Autodesk Inventor part; units mm, degrees
(part 10 of 15)
  arc A4366 (-10.816, -104.5572) -> (-10.816, -104.6588) centre (-10.816, -104.608) ccw
  arc A4367 (-8.784, -104.6588) -> (-8.784, -104.5572) centre (-8.784, -104.608) ccw
  line L2010 (-10.816, -104.608) -> (-10.816, -103.592)
  arc A4368 (-10.7652, -103.592) -> (-10.8668, -103.592) centre (-10.816, -103.592) ccw
  arc A4369 (-10.8668, -104.608) -> (-10.7652, -104.608) centre (-10.816, -104.608) ccw
  line L2011 (7.584, -84.992) -> (9.616, -84.992)
  arc A4370 (9.616, -85.0428) -> (9.616, -84.9412) centre (9.616, -84.992) ccw
  arc A4371 (7.584, -84.9412) -> (7.584, -85.0428) centre (7.584, -84.992) ccw
  line L2012 (9.616, -84.992) -> (9.616, -86.008)
  arc A4372 (9.5652, -86.008) -> (9.6668, -86.008) centre (9.616, -86.008) ccw
  arc A4373 (9.6668, -84.992) -> (9.5652, -84.992) centre (9.616, -84.992) ccw
  line L2013 (9.616, -86.008) -> (7.584, -86.008)
  arc A4374 (7.584, -85.9572) -> (7.584, -86.0588) centre (7.584, -86.008) ccw
  arc A4375 (9.616, -86.0588) -> (9.616, -85.9572) centre (9.616, -86.008) ccw
  line L2014 (7.584, -86.008) -> (7.584, -84.992)
  arc A4376 (7.6348, -84.992) -> (7.5332, -84.992) centre (7.584, -84.992) ccw
  arc A4377 (7.5332, -86.008) -> (7.6348, -86.008) centre (7.584, -86.008) ccw
  line L2015 (-8.416, -105.092) -> (-6.384, -105.092)
  arc A4378 (-6.384, -105.1428) -> (-6.384, -105.0412) centre (-6.384, -105.092) ccw
  arc A4379 (-8.416, -105.0412) -> (-8.416, -105.1428) centre (-8.416, -105.092) ccw
  line L2016 (-6.384, -105.092) -> (-6.384, -106.108)
  arc A4380 (-6.4348, -106.108) -> (-6.3332, -106.108) centre (-6.384, -106.108) ccw
  arc A4381 (-6.3332, -105.092) -> (-6.4348, -105.092) centre (-6.384, -105.092) ccw
  line L2017 (-6.384, -106.108) -> (-8.416, -106.108)
  arc A4382 (-8.416, -106.0572) -> (-8.416, -106.1588) centre (-8.416, -106.108) ccw
  arc A4383 (-6.384, -106.1588) -> (-6.384, -106.0572) centre (-6.384, -106.108) ccw
  line L2018 (-8.416, -106.108) -> (-8.416, -105.092)
  arc A4384 (-8.3652, -105.092) -> (-8.4668, -105.092) centre (-8.416, -105.092) ccw
  arc A4385 (-8.4668, -106.108) -> (-8.3652, -106.108) centre (-8.416, -106.108) ccw
  line L2019 (-8.416, -107.092) -> (-6.384, -107.092)
  arc A4386 (-6.384, -107.1428) -> (-6.384, -107.0412) centre (-6.384, -107.092) ccw
  arc A4387 (-8.416, -107.0412) -> (-8.416, -107.1428) centre (-8.416, -107.092) ccw
  line L2020 (-6.384, -107.092) -> (-6.384, -108.108)
  arc A4388 (-6.4348, -108.108) -> (-6.3332, -108.108) centre (-6.384, -108.108) ccw
  arc A4389 (-6.3332, -107.092) -> (-6.4348, -107.092) centre (-6.384, -107.092) ccw
  line L2021 (-6.384, -108.108) -> (-8.416, -108.108)
  arc A4390 (-8.416, -108.0572) -> (-8.416, -108.1588) centre (-8.416, -108.108) ccw
  arc A4391 (-6.384, -108.1588) -> (-6.384, -108.0572) centre (-6.384, -108.108) ccw
  line L2022 (-8.416, -108.108) -> (-8.416, -107.092)
  arc A4392 (-8.3652, -107.092) -> (-8.4668, -107.092) centre (-8.416, -107.092) ccw
  arc A4393 (-8.4668, -108.108) -> (-8.3652, -108.108) centre (-8.416, -108.108) ccw
  line L2023 (7.192, -93.816) -> (7.192, -91.784)
  arc A4394 (7.2428, -91.784) -> (7.1412, -91.784) centre (7.192, -91.784) ccw
  arc A4395 (7.1412, -93.816) -> (7.2428, -93.816) centre (7.192, -93.816) ccw
  line L2024 (7.192, -91.784) -> (8.208, -91.784)
  arc A4396 (8.208, -91.8348) -> (8.208, -91.7332) centre (8.208, -91.784) ccw
  arc A4397 (7.192, -91.7332) -> (7.192, -91.8348) centre (7.192, -91.784) ccw
  line L2025 (8.208, -91.784) -> (8.208, -93.816)
  arc A4398 (8.1572, -93.816) -> (8.2588, -93.816) centre (8.208, -93.816) ccw
  arc A4399 (8.2588, -91.784) -> (8.1572, -91.784) centre (8.208, -91.784) ccw
  line L2026 (8.208, -93.816) -> (7.192, -93.816)
  arc A4400 (7.192, -93.7652) -> (7.192, -93.8668) centre (7.192, -93.816) ccw
  arc A4401 (8.208, -93.8668) -> (8.208, -93.7652) centre (8.208, -93.816) ccw
  line L2027 (-8.416, -108.092) -> (-6.384, -108.092)
  arc A4402 (-6.384, -108.1428) -> (-6.384, -108.0412) centre (-6.384, -108.092) ccw
  arc A4403 (-8.416, -108.0412) -> (-8.416, -108.1428) centre (-8.416, -108.092) ccw
  line L2028 (-6.384, -108.092) -> (-6.384, -109.108)
  arc A4404 (-6.4348, -109.108) -> (-6.3332, -109.108) centre (-6.384, -109.108) ccw
  arc A4405 (-6.3332, -108.092) -> (-6.4348, -108.092) centre (-6.384, -108.092) ccw
  line L2029 (-6.384, -109.108) -> (-8.416, -109.108)
  arc A4406 (-8.416, -109.0572) -> (-8.416, -109.1588) centre (-8.416, -109.108) ccw
  arc A4407 (-6.384, -109.1588) -> (-6.384, -109.0572) centre (-6.384, -109.108) ccw
  line L2030 (-8.416, -109.108) -> (-8.416, -108.092)
  arc A4408 (-8.3652, -108.092) -> (-8.4668, -108.092) centre (-8.416, -108.092) ccw
  arc A4409 (-8.4668, -109.108) -> (-8.3652, -109.108) centre (-8.416, -109.108) ccw
  line L2031 (14.184, -101.792) -> (16.216, -101.792)
  arc A4410 (16.216, -101.8428) -> (16.216, -101.7412) centre (16.216, -101.792) ccw
  arc A4411 (14.184, -101.7412) -> (14.184, -101.8428) centre (14.184, -101.792) ccw
  line L2032 (16.216, -101.792) -> (16.216, -102.808)
  arc A4412 (16.1652, -102.808) -> (16.2668, -102.808) centre (16.216, -102.808) ccw
  arc A4413 (16.2668, -101.792) -> (16.1652, -101.792) centre (16.216, -101.792) ccw
  line L2033 (16.216, -102.808) -> (14.184, -102.808)
  arc A4414 (14.184, -102.7572) -> (14.184, -102.8588) centre (14.184, -102.808) ccw
  arc A4415 (16.216, -102.8588) -> (16.216, -102.7572) centre (16.216, -102.808) ccw
  line L2034 (14.184, -102.808) -> (14.184, -101.792)
  arc A4416 (14.2348, -101.792) -> (14.1332, -101.792) centre (14.184, -101.792) ccw
  arc A4417 (14.1332, -102.808) -> (14.2348, -102.808) centre (14.184, -102.808) ccw
  line L2035 (12.184, -103.792) -> (14.216, -103.792)
  arc A4418 (14.216, -103.8428) -> (14.216, -103.7412) centre (14.216, -103.792) ccw
  arc A4419 (12.184, -103.7412) -> (12.184, -103.8428) centre (12.184, -103.792) ccw
  line L2036 (14.216, -103.792) -> (14.216, -104.808)
  arc A4420 (14.1652, -104.808) -> (14.2668, -104.808) centre (14.216, -104.808) ccw
  arc A4421 (14.2668, -103.792) -> (14.1652, -103.792) centre (14.216, -103.792) ccw
  line L2037 (14.216, -104.808) -> (12.184, -104.808)
  arc A4422 (12.184, -104.7572) -> (12.184, -104.8588) centre (12.184, -104.808) ccw
  arc A4423 (14.216, -104.8588) -> (14.216, -104.7572) centre (14.216, -104.808) ccw
  line L2038 (12.184, -104.808) -> (12.184, -103.792)
  arc A4424 (12.2348, -103.792) -> (12.1332, -103.792) centre (12.184, -103.792) ccw
  arc A4425 (12.1332, -104.808) -> (12.2348, -104.808) centre (12.184, -104.808) ccw
  line L2039 (10.316, -91.608) -> (8.284, -91.608)
  arc A4426 (8.284, -91.5572) -> (8.284, -91.6588) centre (8.284, -91.608) ccw
  arc A4427 (10.316, -91.6588) -> (10.316, -91.5572) centre (10.316, -91.608) ccw
  line L2040 (8.284, -91.608) -> (8.284, -90.592)
  arc A4428 (8.3348, -90.592) -> (8.2332, -90.592) centre (8.284, -90.592) ccw
  arc A4429 (8.2332, -91.608) -> (8.3348, -91.608) centre (8.284, -91.608) ccw
  line L2041 (8.284, -90.592) -> (10.316, -90.592)
  arc A4430 (10.316, -90.6428) -> (10.316, -90.5412) centre (10.316, -90.592) ccw
  arc A4431 (8.284, -90.5412) -> (8.284, -90.6428) centre (8.284, -90.592) ccw
  line L2042 (10.316, -90.592) -> (10.316, -91.608)
  arc A4432 (10.2652, -91.608) -> (10.3668, -91.608) centre (10.316, -91.608) ccw
  arc A4433 (10.3668, -90.592) -> (10.2652, -90.592) centre (10.316, -90.592) ccw
  line L2043 (12.208, -101.784) -> (12.208, -103.816)
  arc A4434 (12.1572, -103.816) -> (12.2588, -103.816) centre (12.208, -103.816) ccw
  arc A4435 (12.2588, -101.784) -> (12.1572, -101.784) centre (12.208, -101.784) ccw
  line L2044 (12.208, -103.816) -> (11.192, -103.816)
  arc A4436 (11.192, -103.7652) -> (11.192, -103.8668) centre (11.192, -103.816) ccw
  arc A4437 (12.208, -103.8668) -> (12.208, -103.7652) centre (12.208, -103.816) ccw
  line L2045 (11.192, -103.816) -> (11.192, -101.784)
  arc A4438 (11.2428, -101.784) -> (11.1412, -101.784) centre (11.192, -101.784) ccw
  arc A4439 (11.1412, -103.816) -> (11.2428, -103.816) centre (11.192, -103.816) ccw
  line L2046 (11.192, -101.784) -> (12.208, -101.784)
  arc A4440 (12.208, -101.8348) -> (12.208, -101.7332) centre (12.208, -101.784) ccw
  arc A4441 (11.192, -101.7332) -> (11.192, -101.8348) centre (11.192, -101.784) ccw
  line L2047 (-5.416, -107.092) -> (-3.384, -107.092)
  arc A4442 (-3.384, -107.1428) -> (-3.384, -107.0412) centre (-3.384, -107.092) ccw
  arc A4443 (-5.416, -107.0412) -> (-5.416, -107.1428) centre (-5.416, -107.092) ccw
  line L2048 (-3.384, -107.092) -> (-3.384, -108.108)
  arc A4444 (-3.4348, -108.108) -> (-3.3332, -108.108) centre (-3.384, -108.108) ccw
  arc A4445 (-3.3332, -107.092) -> (-3.4348, -107.092) centre (-3.384, -107.092) ccw
  line L2049 (-3.384, -108.108) -> (-5.416, -108.108)
  arc A4446 (-5.416, -108.0572) -> (-5.416, -108.1588) centre (-5.416, -108.108) ccw
  arc A4447 (-3.384, -108.1588) -> (-3.384, -108.0572) centre (-3.384, -108.108) ccw
  line L2050 (-5.416, -108.108) -> (-5.416, -107.092)
  arc A4448 (-5.3652, -107.092) -> (-5.4668, -107.092) centre (-5.416, -107.092) ccw
  arc A4449 (-5.4668, -108.108) -> (-5.3652, -108.108) centre (-5.416, -108.108) ccw
  line L2051 (14.184, -103.792) -> (16.216, -103.792)
  arc A4450 (16.216, -103.8428) -> (16.216, -103.7412) centre (16.216, -103.792) ccw
  arc A4451 (14.184, -103.7412) -> (14.184, -103.8428) centre (14.184, -103.792) ccw
  line L2052 (16.216, -103.792) -> (16.216, -104.808)
  arc A4452 (16.1652, -104.808) -> (16.2668, -104.808) centre (16.216, -104.808) ccw
  arc A4453 (16.2668, -103.792) -> (16.1652, -103.792) centre (16.216, -103.792) ccw
  line L2053 (16.216, -104.808) -> (14.184, -104.808)
  arc A4454 (14.184, -104.7572) -> (14.184, -104.8588) centre (14.184, -104.808) ccw
  arc A4455 (16.216, -104.8588) -> (16.216, -104.7572) centre (16.216, -104.808) ccw
  line L2054 (14.184, -104.808) -> (14.184, -103.792)
  arc A4456 (14.2348, -103.792) -> (14.1332, -103.792) centre (14.184, -103.792) ccw
  arc A4457 (14.1332, -104.808) -> (14.2348, -104.808) centre (14.184, -104.808) ccw
  line L2055 (14.208, -101.784) -> (14.208, -103.816)
  arc A4458 (14.1572, -103.816) -> (14.2588, -103.816) centre (14.208, -103.816) ccw
  arc A4459 (14.2588, -101.784) -> (14.1572, -101.784) centre (14.208, -101.784) ccw
  line L2056 (14.208, -103.816) -> (13.192, -103.816)
  arc A4460 (13.192, -103.7652) -> (13.192, -103.8668) centre (13.192, -103.816) ccw
  arc A4461 (14.208, -103.8668) -> (14.208, -103.7652) centre (14.208, -103.816) ccw
  line L2057 (13.192, -103.816) -> (13.192, -101.784)
  arc A4462 (13.2428, -101.784) -> (13.1412, -101.784) centre (13.192, -101.784) ccw
  arc A4463 (13.1412, -103.816) -> (13.2428, -103.816) centre (13.192, -103.816) ccw
  line L2058 (13.192, -101.784) -> (14.208, -101.784)
  arc A4464 (14.208, -101.8348) -> (14.208, -101.7332) centre (14.208, -101.784) ccw
  arc A4465 (13.192, -101.7332) -> (13.192, -101.8348) centre (13.192, -101.784) ccw
  line L2059 (-6.916, 46.508) -> (-4.884, 46.508)
  arc A4466 (-4.884, 46.4572) -> (-4.884, 46.5588) centre (-4.884, 46.508) ccw
  arc A4467 (-6.916, 46.5588) -> (-6.916, 46.4572) centre (-6.916, 46.508) ccw
  line L2060 (-4.884, 46.508) -> (-4.884, 45.492)
  arc A4468 (-4.9348, 45.492) -> (-4.8332, 45.492) centre (-4.884, 45.492) ccw
  arc A4469 (-4.8332, 46.508) -> (-4.9348, 46.508) centre (-4.884, 46.508) ccw
  line L2061 (-4.884, 45.492) -> (-6.916, 45.492)
  arc A4470 (-6.916, 45.5428) -> (-6.916, 45.4412) centre (-6.916, 45.492) ccw
  arc A4471 (-4.884, 45.4412) -> (-4.884, 45.5428) centre (-4.884, 45.492) ccw
  line L2062 (-6.916, 45.492) -> (-6.916, 46.508)
  arc A4472 (-6.8652, 46.508) -> (-6.9668, 46.508) centre (-6.916, 46.508) ccw
  arc A4473 (-6.9668, 45.492) -> (-6.8652, 45.492) centre (-6.916, 45.492) ccw
  line L2063 (-6.392, 38.216) -> (-6.392, 36.184)
  arc A4474 (-6.4428, 36.184) -> (-6.3412, 36.184) centre (-6.392, 36.184) ccw
  arc A4475 (-6.3412, 38.216) -> (-6.4428, 38.216) centre (-6.392, 38.216) ccw
  line L2064 (-6.392, 36.184) -> (-7.408, 36.184)
  arc A4476 (-7.408, 36.2348) -> (-7.408, 36.1332) centre (-7.408, 36.184) ccw
  arc A4477 (-6.392, 36.1332) -> (-6.392, 36.2348) centre (-6.392, 36.184) ccw
  line L2065 (-7.408, 36.184) -> (-7.408, 38.216)
  arc A4478 (-7.3572, 38.216) -> (-7.4588, 38.216) centre (-7.408, 38.216) ccw
  arc A4479 (-7.4588, 36.184) -> (-7.3572, 36.184) centre (-7.408, 36.184) ccw
  line L2066 (-7.408, 38.216) -> (-6.392, 38.216)
  arc A4480 (-6.392, 38.1652) -> (-6.392, 38.2668) centre (-6.392, 38.216) ccw
  arc A4481 (-7.408, 38.2668) -> (-7.408, 38.1652) centre (-7.408, 38.216) ccw
  line L2067 (-7.392, 38.216) -> (-7.392, 36.184)
  arc A4482 (-7.4428, 36.184) -> (-7.3412, 36.184) centre (-7.392, 36.184) ccw
  arc A4483 (-7.3412, 38.216) -> (-7.4428, 38.216) centre (-7.392, 38.216) ccw
  line L2068 (-7.392, 36.184) -> (-8.408, 36.184)
  arc A4484 (-8.408, 36.2348) -> (-8.408, 36.1332) centre (-8.408, 36.184) ccw
  arc A4485 (-7.392, 36.1332) -> (-7.392, 36.2348) centre (-7.392, 36.184) ccw
  line L2069 (-8.408, 36.184) -> (-8.408, 38.216)
  arc A4486 (-8.3572, 38.216) -> (-8.4588, 38.216) centre (-8.408, 38.216) ccw
  arc A4487 (-8.4588, 36.184) -> (-8.3572, 36.184) centre (-8.408, 36.184) ccw
  line L2070 (-8.408, 38.216) -> (-7.392, 38.216)
  arc A4488 (-7.392, 38.1652) -> (-7.392, 38.2668) centre (-7.392, 38.216) ccw
  arc A4489 (-8.408, 38.2668) -> (-8.408, 38.1652) centre (-8.408, 38.216) ccw
  line L2071 (-4.016, 39.308) -> (-1.984, 39.308)
  arc A4490 (-1.984, 39.2572) -> (-1.984, 39.3588) centre (-1.984, 39.308) ccw
  arc A4491 (-4.016, 39.3588) -> (-4.016, 39.2572) centre (-4.016, 39.308) ccw
  line L2072 (-1.984, 39.308) -> (-1.984, 38.292)
  arc A4492 (-2.0348, 38.292) -> (-1.9332, 38.292) centre (-1.984, 38.292) ccw
  arc A4493 (-1.9332, 39.308) -> (-2.0348, 39.308) centre (-1.984, 39.308) ccw
  line L2073 (-1.984, 38.292) -> (-4.016, 38.292)
  arc A4494 (-4.016, 38.3428) -> (-4.016, 38.2412) centre (-4.016, 38.292) ccw
  arc A4495 (-1.984, 38.2412) -> (-1.984, 38.3428) centre (-1.984, 38.292) ccw
  line L2074 (-4.016, 38.292) -> (-4.016, 39.308)
  arc A4496 (-3.9652, 39.308) -> (-4.0668, 39.308) centre (-4.016, 39.308) ccw
  arc A4497 (-4.0668, 38.292) -> (-3.9652, 38.292) centre (-4.016, 38.292) ccw
  line L2075 (-9.484, 40.892) -> (-11.516, 40.892)
  arc A4498 (-11.516, 40.9428) -> (-11.516, 40.8412) centre (-11.516, 40.892) ccw
  arc A4499 (-9.484, 40.8412) -> (-9.484, 40.9428) centre (-9.484, 40.892) ccw
  line L2076 (-11.516, 40.892) -> (-11.516, 41.908)
  arc A4500 (-11.4652, 41.908) -> (-11.5668, 41.908) centre (-11.516, 41.908) ccw
  arc A4501 (-11.5668, 40.892) -> (-11.4652, 40.892) centre (-11.516, 40.892) ccw
  line L2077 (-11.516, 41.908) -> (-9.484, 41.908)
  arc A4502 (-9.484, 41.8572) -> (-9.484, 41.9588) centre (-9.484, 41.908) ccw
  arc A4503 (-11.516, 41.9588) -> (-11.516, 41.8572) centre (-11.516, 41.908) ccw
  line L2078 (-9.484, 41.908) -> (-9.484, 40.892)
  arc A4504 (-9.5348, 40.892) -> (-9.4332, 40.892) centre (-9.484, 40.892) ccw
  arc A4505 (-9.4332, 41.908) -> (-9.5348, 41.908) centre (-9.484, 41.908) ccw
  line L2079 (-4.884, 44.492) -> (-6.916, 44.492)
  arc A4506 (-6.916, 44.5428) -> (-6.916, 44.4412) centre (-6.916, 44.492) ccw
  arc A4507 (-4.884, 44.4412) -> (-4.884, 44.5428) centre (-4.884, 44.492) ccw
  line L2080 (-6.916, 44.492) -> (-6.916, 45.508)
  arc A4508 (-6.8652, 45.508) -> (-6.9668, 45.508) centre (-6.916, 45.508) ccw
  arc A4509 (-6.9668, 44.492) -> (-6.8652, 44.492) centre (-6.916, 44.492) ccw
  line L2081 (-6.916, 45.508) -> (-4.884, 45.508)
  arc A4510 (-4.884, 45.4572) -> (-4.884, 45.5588) centre (-4.884, 45.508) ccw
  arc A4511 (-6.916, 45.5588) -> (-6.916, 45.4572) centre (-6.916, 45.508) ccw
  line L2082 (-4.884, 45.508) -> (-4.884, 44.492)
  arc A4512 (-4.9348, 44.492) -> (-4.8332, 44.492) centre (-4.884, 44.492) ccw
  arc A4513 (-4.8332, 45.508) -> (-4.9348, 45.508) centre (-4.884, 45.508) ccw
  line L2083 (-1.392, -88.984) -> (-1.392, -91.016)
  arc A4514 (-1.4428, -91.016) -> (-1.3412, -91.016) centre (-1.392, -91.016) ccw
  arc A4515 (-1.3412, -88.984) -> (-1.4428, -88.984) centre (-1.392, -88.984) ccw
  line L2084 (-1.392, -91.016) -> (-2.408, -91.016)
  arc A4516 (-2.408, -90.9652) -> (-2.408, -91.0668) centre (-2.408, -91.016) ccw
  arc A4517 (-1.392, -91.0668) -> (-1.392, -90.9652) centre (-1.392, -91.016) ccw
  line L2085 (-2.408, -91.016) -> (-2.408, -88.984)
  arc A4518 (-2.3572, -88.984) -> (-2.4588, -88.984) centre (-2.408, -88.984) ccw
  arc A4519 (-2.4588, -91.016) -> (-2.3572, -91.016) centre (-2.408, -91.016) ccw
  line L2086 (-2.408, -88.984) -> (-1.392, -88.984)
  arc A4520 (-1.392, -89.0348) -> (-1.392, -88.9332) centre (-1.392, -88.984) ccw
  arc A4521 (-2.408, -88.9332) -> (-2.408, -89.0348) centre (-2.408, -88.984) ccw
  line L2087 (16.284, -83.392) -> (18.316, -83.392)
  arc A4522 (18.316, -83.4428) -> (18.316, -83.3412) centre (18.316, -83.392) ccw
  arc A4523 (16.284, -83.3412) -> (16.284, -83.4428) centre (16.284, -83.392) ccw
  line L2088 (18.316, -83.392) -> (18.316, -84.408)
  arc A4524 (18.2652, -84.408) -> (18.3668, -84.408) centre (18.316, -84.408) ccw
  arc A4525 (18.3668, -83.392) -> (18.2652, -83.392) centre (18.316, -83.392) ccw
  line L2089 (18.316, -84.408) -> (16.284, -84.408)
  arc A4526 (16.284, -84.3572) -> (16.284, -84.4588) centre (16.284, -84.408) ccw
  arc A4527 (18.316, -84.4588) -> (18.316, -84.3572) centre (18.316, -84.408) ccw
  line L2090 (16.284, -84.408) -> (16.284, -83.392)
  arc A4528 (16.3348, -83.392) -> (16.2332, -83.392) centre (16.284, -83.392) ccw
  arc A4529 (16.2332, -84.408) -> (16.3348, -84.408) centre (16.284, -84.408) ccw
  line L2091 (-21.992, -6.784) -> (-21.992, -8.816)
  arc A4530 (-22.0428, -8.816) -> (-21.9412, -8.816) centre (-21.992, -8.816) ccw
  arc A4531 (-21.9412, -6.784) -> (-22.0428, -6.784) centre (-21.992, -6.784) ccw
  line L2092 (-21.992, -8.816) -> (-23.008, -8.816)
  arc A4532 (-23.008, -8.7652) -> (-23.008, -8.8668) centre (-23.008, -8.816) ccw
  arc A4533 (-21.992, -8.8668) -> (-21.992, -8.7652) centre (-21.992, -8.816) ccw
  line L2093 (-23.008, -8.816) -> (-23.008, -6.784)
  arc A4534 (-22.9572, -6.784) -> (-23.0588, -6.784) centre (-23.008, -6.784) ccw
  arc A4535 (-23.0588, -8.816) -> (-22.9572, -8.816) centre (-23.008, -8.816) ccw
  line L2094 (-23.008, -6.784) -> (-21.992, -6.784)
  arc A4536 (-21.992, -6.8348) -> (-21.992, -6.7332) centre (-21.992, -6.784) ccw
  arc A4537 (-23.008, -6.7332) -> (-23.008, -6.8348) centre (-23.008, -6.784) ccw
  line L2095 (-16.992, 16.216) -> (-16.992, 14.184)
  arc A4538 (-17.0428, 14.184) -> (-16.9412, 14.184) centre (-16.992, 14.184) ccw
  arc A4539 (-16.9412, 16.216) -> (-17.0428, 16.216) centre (-16.992, 16.216) ccw
  line L2096 (-16.992, 14.184) -> (-18.008, 14.184)
  arc A4540 (-18.008, 14.2348) -> (-18.008, 14.1332) centre (-18.008, 14.184) ccw
  arc A4541 (-16.992, 14.1332) -> (-16.992, 14.2348) centre (-16.992, 14.184) ccw
  line L2097 (-18.008, 14.184) -> (-18.008, 16.216)
  arc A4542 (-17.9572, 16.216) -> (-18.0588, 16.216) centre (-18.008, 16.216) ccw
  arc A4543 (-18.0588, 14.184) -> (-17.9572, 14.184) centre (-18.008, 14.184) ccw
  line L2098 (-18.008, 16.216) -> (-16.992, 16.216)
  arc A4544 (-16.992, 16.1652) -> (-16.992, 16.2668) centre (-16.992, 16.216) ccw
  arc A4545 (-18.008, 16.2668) -> (-18.008, 16.1652) centre (-18.008, 16.216) ccw
  line L2099 (-9.992, 8.216) -> (-9.992, 6.184)
  arc A4546 (-10.0428, 6.184) -> (-9.9412, 6.184) centre (-9.992, 6.184) ccw
  arc A4547 (-9.9412, 8.216) -> (-10.0428, 8.216) centre (-9.992, 8.216) ccw
  line L2100 (-9.992, 6.184) -> (-11.008, 6.184)
  arc A4548 (-11.008, 6.2348) -> (-11.008, 6.1332) centre (-11.008, 6.184) ccw
  arc A4549 (-9.992, 6.1332) -> (-9.992, 6.2348) centre (-9.992, 6.184) ccw
  line L2101 (-11.008, 6.184) -> (-11.008, 8.216)
  arc A4550 (-10.9572, 8.216) -> (-11.0588, 8.216) centre (-11.008, 8.216) ccw
  arc A4551 (-11.0588, 6.184) -> (-10.9572, 6.184) centre (-11.008, 6.184) ccw
  line L2102 (-11.008, 8.216) -> (-9.992, 8.216)
  arc A4552 (-9.992, 8.1652) -> (-9.992, 8.2668) centre (-9.992, 8.216) ccw
  arc A4553 (-11.008, 8.2668) -> (-11.008, 8.1652) centre (-11.008, 8.216) ccw
  line L2103 (1.008, 10.216) -> (1.008, 8.184)
  arc A4554 (0.9572, 8.184) -> (1.0588, 8.184) centre (1.008, 8.184) ccw
  arc A4555 (1.0588, 10.216) -> (0.9572, 10.216) centre (1.008, 10.216) ccw
  line L2104 (1.008, 8.184) -> (-0.008, 8.184)
  arc A4556 (-0.008, 8.2348) -> (-0.008, 8.1332) centre (-0.008, 8.184) ccw
  arc A4557 (1.008, 8.1332) -> (1.008, 8.2348) centre (1.008, 8.184) ccw
  line L2105 (-0.008, 8.184) -> (-0.008, 10.216)
  arc A4558 (0.0428, 10.216) -> (-0.0588, 10.216) centre (-0.008, 10.216) ccw
  arc A4559 (-0.0588, 8.184) -> (0.0428, 8.184) centre (-0.008, 8.184) ccw
  line L2106 (-0.008, 10.216) -> (1.008, 10.216)
  arc A4560 (1.008, 10.1652) -> (1.008, 10.2668) centre (1.008, 10.216) ccw
  arc A4561 (-0.008, 10.2668) -> (-0.008, 10.1652) centre (-0.008, 10.216) ccw
  line L2107 (-0.008, 10.184) -> (-0.008, 12.216)
  arc A4562 (0.0428, 12.216) -> (-0.0588, 12.216) centre (-0.008, 12.216) ccw
  arc A4563 (-0.0588, 10.184) -> (0.0428, 10.184) centre (-0.008, 10.184) ccw
  line L2108 (-0.008, 12.216) -> (1.008, 12.216)
  arc A4564 (1.008, 12.1652) -> (1.008, 12.2668) centre (1.008, 12.216) ccw
  arc A4565 (-0.008, 12.2668) -> (-0.008, 12.1652) centre (-0.008, 12.216) ccw
  line L2109 (1.008, 12.216) -> (1.008, 10.184)
  arc A4566 (0.9572, 10.184) -> (1.0588, 10.184) centre (1.008, 10.184) ccw
  arc A4567 (1.0588, 12.216) -> (0.9572, 12.216) centre (1.008, 12.216) ccw
  line L2110 (1.008, 10.184) -> (-0.008, 10.184)
  arc A4568 (-0.008, 10.2348) -> (-0.008, 10.1332) centre (-0.008, 10.184) ccw
  arc A4569 (1.008, 10.1332) -> (1.008, 10.2348) centre (1.008, 10.184) ccw
  line L2111 (6.016, 10.192) -> (3.984, 10.192)
  arc A4570 (3.984, 10.2428) -> (3.984, 10.1412) centre (3.984, 10.192) ccw
  arc A4571 (6.016, 10.1412) -> (6.016, 10.2428) centre (6.016, 10.192) ccw
  line L2112 (3.984, 10.192) -> (3.984, 11.208)
  arc A4572 (4.0348, 11.208) -> (3.9332, 11.208) centre (3.984, 11.208) ccw
  arc A4573 (3.9332, 10.192) -> (4.0348, 10.192) centre (3.984, 10.192) ccw
  line L2113 (3.984, 11.208) -> (6.016, 11.208)
  arc A4574 (6.016, 11.1572) -> (6.016, 11.2588) centre (6.016, 11.208) ccw
  arc A4575 (3.984, 11.2588) -> (3.984, 11.1572) centre (3.984, 11.208) ccw
  line L2114 (6.016, 11.208) -> (6.016, 10.192)
  arc A4576 (5.9652, 10.192) -> (6.0668, 10.192) centre (6.016, 10.192) ccw
  arc A4577 (6.0668, 11.208) -> (5.9652, 11.208) centre (6.016, 11.208) ccw
  line L2115 (-0.984, 0.192) -> (-3.016, 0.192)
  arc A4578 (-3.016, 0.2428) -> (-3.016, 0.1412) centre (-3.016, 0.192) ccw
  arc A4579 (-0.984, 0.1412) -> (-0.984, 0.2428) centre (-0.984, 0.192) ccw
  line L2116 (-3.016, 0.192) -> (-3.016, 1.208)
  arc A4580 (-2.9652, 1.208) -> (-3.0668, 1.208) centre (-3.016, 1.208) ccw
  arc A4581 (-3.0668, 0.192) -> (-2.9652, 0.192) centre (-3.016, 0.192) ccw
  line L2117 (-3.016, 1.208) -> (-0.984, 1.208)
  arc A4582 (-0.984, 1.1572) -> (-0.984, 1.2588) centre (-0.984, 1.208) ccw
  arc A4583 (-3.016, 1.2588) -> (-3.016, 1.1572) centre (-3.016, 1.208) ccw
  line L2118 (-0.984, 1.208) -> (-0.984, 0.192)
  arc A4584 (-1.0348, 0.192) -> (-0.9332, 0.192) centre (-0.984, 0.192) ccw
  arc A4585 (-0.9332, 1.208) -> (-1.0348, 1.208) centre (-0.984, 1.208) ccw
  line L2119 (-2.008, -6.816) -> (-2.008, -4.784)
  arc A4586 (-1.9572, -4.784) -> (-2.0588, -4.784) centre (-2.008, -4.784) ccw
  arc A4587 (-2.0588, -6.816) -> (-1.9572, -6.816) centre (-2.008, -6.816) ccw
  line L2120 (-2.008, -4.784) -> (-0.992, -4.784)
  arc A4588 (-0.992, -4.8348) -> (-0.992, -4.7332) centre (-0.992, -4.784) ccw
  arc A4589 (-2.008, -4.7332) -> (-2.008, -4.8348) centre (-2.008, -4.784) ccw
  line L2121 (-0.992, -4.784) -> (-0.992, -6.816)
  arc A4590 (-1.0428, -6.816) -> (-0.9412, -6.816) centre (-0.992, -6.816) ccw
  arc A4591 (-0.9412, -4.784) -> (-1.0428, -4.784) centre (-0.992, -4.784) ccw
  line L2122 (-0.992, -6.816) -> (-2.008, -6.816)
  arc A4592 (-2.008, -6.7652) -> (-2.008, -6.8668) centre (-2.008, -6.816) ccw
  arc A4593 (-0.992, -6.8668) -> (-0.992, -6.7652) centre (-0.992, -6.816) ccw
  line L2123 (1.016, 7.192) -> (-1.016, 7.192)
  arc A4594 (-1.016, 7.2428) -> (-1.016, 7.1412) centre (-1.016, 7.192) ccw
  arc A4595 (1.016, 7.1412) -> (1.016, 7.2428) centre (1.016, 7.192) ccw
  line L2124 (-1.016, 7.192) -> (-1.016, 8.208)
  arc A4596 (-0.9652, 8.208) -> (-1.0668, 8.208) centre (-1.016, 8.208) ccw
  arc A4597 (-1.0668, 7.192) -> (-0.9652, 7.192) centre (-1.016, 7.192) ccw
  line L2125 (-1.016, 8.208) -> (1.016, 8.208)
  arc A4598 (1.016, 8.1572) -> (1.016, 8.2588) centre (1.016, 8.208) ccw
  arc A4599 (-1.016, 8.2588) -> (-1.016, 8.1572) centre (-1.016, 8.208) ccw
  line L2126 (1.016, 8.208) -> (1.016, 7.192)
  arc A4600 (0.9652, 7.192) -> (1.0668, 7.192) centre (1.016, 7.192) ccw
  arc A4601 (1.0668, 8.208) -> (0.9652, 8.208) centre (1.016, 8.208) ccw
  line L2127 (2.008, 9.216) -> (2.008, 7.184)
  arc A4602 (1.9572, 7.184) -> (2.0588, 7.184) centre (2.008, 7.184) ccw
  arc A4603 (2.0588, 9.216) -> (1.9572, 9.216) centre (2.008, 9.216) ccw
  line L2128 (2.008, 7.184) -> (0.992, 7.184)
  arc A4604 (0.992, 7.2348) -> (0.992, 7.1332) centre (0.992, 7.184) ccw
  arc A4605 (2.008, 7.1332) -> (2.008, 7.2348) centre (2.008, 7.184) ccw
  line L2129 (0.992, 7.184) -> (0.992, 9.216)
  arc A4606 (1.0428, 9.216) -> (0.9412, 9.216) centre (0.992, 9.216) ccw
  arc A4607 (0.9412, 7.184) -> (1.0428, 7.184) centre (0.992, 7.184) ccw
  line L2130 (0.992, 9.216) -> (2.008, 9.216)
  arc A4608 (2.008, 9.1652) -> (2.008, 9.2668) centre (2.008, 9.216) ccw
  arc A4609 (0.992, 9.2668) -> (0.992, 9.1652) centre (0.992, 9.216) ccw
  line L2131 (-0.016, 7.208) -> (2.016, 7.208)
  arc A4610 (2.016, 7.1572) -> (2.016, 7.2588) centre (2.016, 7.208) ccw
  arc A4611 (-0.016, 7.2588) -> (-0.016, 7.1572) centre (-0.016, 7.208) ccw
  line L2132 (2.016, 7.208) -> (2.016, 6.192)
  arc A4612 (1.9652, 6.192) -> (2.0668, 6.192) centre (2.016, 6.192) ccw
  arc A4613 (2.0668, 7.208) -> (1.9652, 7.208) centre (2.016, 7.208) ccw
  line L2133 (2.016, 6.192) -> (-0.016, 6.192)
  arc A4614 (-0.016, 6.2428) -> (-0.016, 6.1412) centre (-0.016, 6.192) ccw
  arc A4615 (2.016, 6.1412) -> (2.016, 6.2428) centre (2.016, 6.192) ccw
  line L2134 (-0.016, 6.192) -> (-0.016, 7.208)
  arc A4616 (0.0348, 7.208) -> (-0.0668, 7.208) centre (-0.016, 7.208) ccw
  arc A4617 (-0.0668, 6.192) -> (0.0348, 6.192) centre (-0.016, 6.192) ccw
  line L2135 (-1.016, 6.208) -> (1.016, 6.208)
  arc A4618 (1.016, 6.1572) -> (1.016, 6.2588) centre (1.016, 6.208) ccw
  arc A4619 (-1.016, 6.2588) -> (-1.016, 6.1572) centre (-1.016, 6.208) ccw
  line L2136 (1.016, 6.208) -> (1.016, 5.192)
  arc A4620 (0.9652, 5.192) -> (1.0668, 5.192) centre (1.016, 5.192) ccw
  arc A4621 (1.0668, 6.208) -> (0.9652, 6.208) centre (1.016, 6.208) ccw
  line L2137 (1.016, 5.192) -> (-1.016, 5.192)
  arc A4622 (-1.016, 5.2428) -> (-1.016, 5.1412) centre (-1.016, 5.192) ccw
  arc A4623 (1.016, 5.1412) -> (1.016, 5.2428) centre (1.016, 5.192) ccw
  line L2138 (-1.016, 5.192) -> (-1.016, 6.208)
  arc A4624 (-0.9652, 6.208) -> (-1.0668, 6.208) centre (-1.016, 6.208) ccw
  arc A4625 (-1.0668, 5.192) -> (-0.9652, 5.192) centre (-1.016, 5.192) ccw
  line L2139 (-13.892, -20.684) -> (-13.892, -22.716)
  arc A4626 (-13.9428, -22.716) -> (-13.8412, -22.716) centre (-13.892, -22.716) ccw
  arc A4627 (-13.8412, -20.684) -> (-13.9428, -20.684) centre (-13.892, -20.684) ccw
  line L2140 (-13.892, -22.716) -> (-14.908, -22.716)
  arc A4628 (-14.908, -22.6652) -> (-14.908, -22.7668) centre (-14.908, -22.716) ccw
  arc A4629 (-13.892, -22.7668) -> (-13.892, -22.6652) centre (-13.892, -22.716) ccw
  line L2141 (-14.908, -22.716) -> (-14.908, -20.684)
  arc A4630 (-14.8572, -20.684) -> (-14.9588, -20.684) centre (-14.908, -20.684) ccw
  arc A4631 (-14.9588, -22.716) -> (-14.8572, -22.716) centre (-14.908, -22.716) ccw
  line L2142 (-14.908, -20.684) -> (-13.892, -20.684)
  arc A4632 (-13.892, -20.7348) -> (-13.892, -20.6332) centre (-13.892, -20.684) ccw
  arc A4633 (-14.908, -20.6332) -> (-14.908, -20.7348) centre (-14.908, -20.684) ccw
  line L2143 (-7.992, 2.216) -> (-7.992, 0.184)
  arc A4634 (-8.0428, 0.184) -> (-7.9412, 0.184) centre (-7.992, 0.184) ccw
  arc A4635 (-7.9412, 2.216) -> (-8.0428, 2.216) centre (-7.992, 2.216) ccw
  line L2144 (-7.992, 0.184) -> (-9.008, 0.184)
  arc A4636 (-9.008, 0.2348) -> (-9.008, 0.1332) centre (-9.008, 0.184) ccw
  arc A4637 (-7.992, 0.1332) -> (-7.992, 0.2348) centre (-7.992, 0.184) ccw
  line L2145 (-9.008, 0.184) -> (-9.008, 2.216)
  arc A4638 (-8.9572, 2.216) -> (-9.0588, 2.216) centre (-9.008, 2.216) ccw
  arc A4639 (-9.0588, 0.184) -> (-8.9572, 0.184) centre (-9.008, 0.184) ccw
  line L2146 (-9.008, 2.216) -> (-7.992, 2.216)
  arc A4640 (-7.992, 2.1652) -> (-7.992, 2.2668) centre (-7.992, 2.216) ccw
  arc A4641 (-9.008, 2.2668) -> (-9.008, 2.1652) centre (-9.008, 2.216) ccw
  line L2147 (-6.992, 2.216) -> (-6.992, 0.184)
  arc A4642 (-7.0428, 0.184) -> (-6.9412, 0.184) centre (-6.992, 0.184) ccw
  arc A4643 (-6.9412, 2.216) -> (-7.0428, 2.216) centre (-6.992, 2.216) ccw
  line L2148 (-6.992, 0.184) -> (-8.008, 0.184)
  arc A4644 (-8.008, 0.2348) -> (-8.008, 0.1332) centre (-8.008, 0.184) ccw
  arc A4645 (-6.992, 0.1332) -> (-6.992, 0.2348) centre (-6.992, 0.184) ccw
  line L2149 (-8.008, 0.184) -> (-8.008, 2.216)
  arc A4646 (-7.9572, 2.216) -> (-8.0588, 2.216) centre (-8.008, 2.216) ccw
  arc A4647 (-8.0588, 0.184) -> (-7.9572, 0.184) centre (-8.008, 0.184) ccw
  line L2150 (-8.008, 2.216) -> (-6.992, 2.216)
  arc A4648 (-6.992, 2.1652) -> (-6.992, 2.2668) centre (-6.992, 2.216) ccw
  arc A4649 (-8.008, 2.2668) -> (-8.008, 2.1652) centre (-8.008, 2.216) ccw
  line L2151 (-6.008, -4.816) -> (-6.008, -2.784)
  arc A4650 (-5.9572, -2.784) -> (-6.0588, -2.784) centre (-6.008, -2.784) ccw
  arc A4651 (-6.0588, -4.816) -> (-5.9572, -4.816) centre (-6.008, -4.816) ccw
  line L2152 (-6.008, -2.784) -> (-4.992, -2.784)
  arc A4652 (-4.992, -2.8348) -> (-4.992, -2.7332) centre (-4.992, -2.784) ccw
  arc A4653 (-6.008, -2.7332) -> (-6.008, -2.8348) centre (-6.008, -2.784) ccw
  line L2153 (-4.992, -2.784) -> (-4.992, -4.816)
  arc A4654 (-5.0428, -4.816) -> (-4.9412, -4.816) centre (-4.992, -4.816) ccw
  arc A4655 (-4.9412, -2.784) -> (-5.0428, -2.784) centre (-4.992, -2.784) ccw
  line L2154 (-4.992, -4.816) -> (-6.008, -4.816)
  arc A4656 (-6.008, -4.7652) -> (-6.008, -4.8668) centre (-6.008, -4.816) ccw
  arc A4657 (-4.992, -4.8668) -> (-4.992, -4.7652) centre (-4.992, -4.816) ccw
  line L2155 (0.984, 4.208) -> (3.016, 4.208)
  arc A4658 (3.016, 4.1572) -> (3.016, 4.2588) centre (3.016, 4.208) ccw
  arc A4659 (0.984, 4.2588) -> (0.984, 4.1572) centre (0.984, 4.208) ccw
  line L2156 (3.016, 4.208) -> (3.016, 3.192)
  arc A4660 (2.9652, 3.192) -> (3.0668, 3.192) centre (3.016, 3.192) ccw
  arc A4661 (3.0668, 4.208) -> (2.9652, 4.208) centre (3.016, 4.208) ccw
  line L2157 (3.016, 3.192) -> (0.984, 3.192)
  arc A4662 (0.984, 3.2428) -> (0.984, 3.1412) centre (0.984, 3.192) ccw
  arc A4663 (3.016, 3.1412) -> (3.016, 3.2428) centre (3.016, 3.192) ccw
  line L2158 (0.984, 3.192) -> (0.984, 4.208)
  arc A4664 (1.0348, 4.208) -> (0.9332, 4.208) centre (0.984, 4.208) ccw
  arc A4665 (0.9332, 3.192) -> (1.0348, 3.192) centre (0.984, 3.192) ccw
  line L2159 (-1.016, 4.208) -> (1.016, 4.208)
  arc A4666 (1.016, 4.1572) -> (1.016, 4.2588) centre (1.016, 4.208) ccw
  arc A4667 (-1.016, 4.2588) -> (-1.016, 4.1572) centre (-1.016, 4.208) ccw
  line L2160 (1.016, 4.208) -> (1.016, 3.192)
  arc A4668 (0.9652, 3.192) -> (1.0668, 3.192) centre (1.016, 3.192) ccw
  arc A4669 (1.0668, 4.208) -> (0.9652, 4.208) centre (1.016, 4.208) ccw
  line L2161 (1.016, 3.192) -> (-1.016, 3.192)
  arc A4670 (-1.016, 3.2428) -> (-1.016, 3.1412) centre (-1.016, 3.192) ccw
  arc A4671 (1.016, 3.1412) -> (1.016, 3.2428) centre (1.016, 3.192) ccw
  line L2162 (-1.016, 3.192) -> (-1.016, 4.208)
  arc A4672 (-0.9652, 4.208) -> (-1.0668, 4.208) centre (-1.016, 4.208) ccw
  arc A4673 (-1.0668, 3.192) -> (-0.9652, 3.192) centre (-1.016, 3.192) ccw
  line L2163 (-2.992, 2.216) -> (-2.992, 0.184)
  arc A4674 (-3.0428, 0.184) -> (-2.9412, 0.184) centre (-2.992, 0.184) ccw
  arc A4675 (-2.9412, 2.216) -> (-3.0428, 2.216) centre (-2.992, 2.216) ccw
  line L2164 (-2.992, 0.184) -> (-4.008, 0.184)
  arc A4676 (-4.008, 0.2348) -> (-4.008, 0.1332) centre (-4.008, 0.184) ccw
  arc A4677 (-2.992, 0.1332) -> (-2.992, 0.2348) centre (-2.992, 0.184) ccw
  line L2165 (-4.008, 0.184) -> (-4.008, 2.216)
  arc A4678 (-3.9572, 2.216) -> (-4.0588, 2.216) centre (-4.008, 2.216) ccw
  arc A4679 (-4.0588, 0.184) -> (-3.9572, 0.184) centre (-4.008, 0.184) ccw
  line L2166 (-4.008, 2.216) -> (-2.992, 2.216)
  arc A4680 (-2.992, 2.1652) -> (-2.992, 2.2668) centre (-2.992, 2.216) ccw
  arc A4681 (-4.008, 2.2668) -> (-4.008, 2.1652) centre (-4.008, 2.216) ccw
  line L2167 (0.984, 3.208) -> (3.016, 3.208)
  arc A4682 (3.016, 3.1572) -> (3.016, 3.2588) centre (3.016, 3.208) ccw
  arc A4683 (0.984, 3.2588) -> (0.984, 3.1572) centre (0.984, 3.208) ccw
  line L2168 (3.016, 3.208) -> (3.016, 2.192)
  arc A4684 (2.9652, 2.192) -> (3.0668, 2.192) centre (3.016, 2.192) ccw
  arc A4685 (3.0668, 3.208) -> (2.9652, 3.208) centre (3.016, 3.208) ccw
  line L2169 (3.016, 2.192) -> (0.984, 2.192)
  arc A4686 (0.984, 2.2428) -> (0.984, 2.1412) centre (0.984, 2.192) ccw
  arc A4687 (3.016, 2.1412) -> (3.016, 2.2428) centre (3.016, 2.192) ccw
  line L2170 (0.984, 2.192) -> (0.984, 3.208)
  arc A4688 (1.0348, 3.208) -> (0.9332, 3.208) centre (0.984, 3.208) ccw
  arc A4689 (0.9332, 2.192) -> (1.0348, 2.192) centre (0.984, 2.192) ccw
  line L2171 (-1.016, 3.208) -> (1.016, 3.208)
  arc A4690 (1.016, 3.1572) -> (1.016, 3.2588) centre (1.016, 3.208) ccw
  arc A4691 (-1.016, 3.2588) -> (-1.016, 3.1572) centre (-1.016, 3.208) ccw
  line L2172 (1.016, 3.208) -> (1.016, 2.192)
  arc A4692 (0.9652, 2.192) -> (1.0668, 2.192) centre (1.016, 2.192) ccw
  arc A4693 (1.0668, 3.208) -> (0.9652, 3.208) centre (1.016, 3.208) ccw
  line L2173 (1.016, 2.192) -> (-1.016, 2.192)
  arc A4694 (-1.016, 2.2428) -> (-1.016, 2.1412) centre (-1.016, 2.192) ccw
  arc A4695 (1.016, 2.1412) -> (1.016, 2.2428) centre (1.016, 2.192) ccw
  line L2174 (-1.016, 2.192) -> (-1.016, 3.208)
  arc A4696 (-0.9652, 3.208) -> (-1.0668, 3.208) centre (-1.016, 3.208) ccw
  arc A4697 (-1.0668, 2.192) -> (-0.9652, 2.192) centre (-1.016, 2.192) ccw
  line L2175 (-7.008, 0.184) -> (-7.008, 2.216)
  arc A4698 (-6.9572, 2.216) -> (-7.0588, 2.216) centre (-7.008, 2.216) ccw
  arc A4699 (-7.0588, 0.184) -> (-6.9572, 0.184) centre (-7.008, 0.184) ccw
  line L2176 (-7.008, 2.216) -> (-5.992, 2.216)
  arc A4700 (-5.992, 2.1652) -> (-5.992, 2.2668) centre (-5.992, 2.216) ccw
  arc A4701 (-7.008, 2.2668) -> (-7.008, 2.1652) centre (-7.008, 2.216) ccw
  line L2177 (-5.992, 2.216) -> (-5.992, 0.184)
  arc A4702 (-6.0428, 0.184) -> (-5.9412, 0.184) centre (-5.992, 0.184) ccw
  arc A4703 (-5.9412, 2.216) -> (-6.0428, 2.216) centre (-5.992, 2.216) ccw
  line L2178 (-5.992, 0.184) -> (-7.008, 0.184)
  arc A4704 (-7.008, 0.2348) -> (-7.008, 0.1332) centre (-7.008, 0.184) ccw
  arc A4705 (-5.992, 0.1332) -> (-5.992, 0.2348) centre (-5.992, 0.184) ccw
  line L2179 (0.984, 2.208) -> (3.016, 2.208)
  arc A4706 (3.016, 2.1572) -> (3.016, 2.2588) centre (3.016, 2.208) ccw
  arc A4707 (0.984, 2.2588) -> (0.984, 2.1572) centre (0.984, 2.208) ccw
  line L2180 (3.016, 2.208) -> (3.016, 1.192)
  arc A4708 (2.9652, 1.192) -> (3.0668, 1.192) centre (3.016, 1.192) ccw
  arc A4709 (3.0668, 2.208) -> (2.9652, 2.208) centre (3.016, 2.208) ccw
  line L2181 (3.016, 1.192) -> (0.984, 1.192)
  arc A4710 (0.984, 1.2428) -> (0.984, 1.1412) centre (0.984, 1.192) ccw
  arc A4711 (3.016, 1.1412) -> (3.016, 1.2428) centre (3.016, 1.192) ccw
  line L2182 (0.984, 1.192) -> (0.984, 2.208)
  arc A4712 (1.0348, 2.208) -> (0.9332, 2.208) centre (0.984, 2.208) ccw
  arc A4713 (0.9332, 1.192) -> (1.0348, 1.192) centre (0.984, 1.192) ccw
  line L2183 (-1.016, 2.208) -> (1.016, 2.208)
  arc A4714 (1.016, 2.1572) -> (1.016, 2.2588) centre (1.016, 2.208) ccw
  arc A4715 (-1.016, 2.2588) -> (-1.016, 2.1572) centre (-1.016, 2.208) ccw
  line L2184 (1.016, 2.208) -> (1.016, 1.192)
  arc A4716 (0.9652, 1.192) -> (1.0668, 1.192) centre (1.016, 1.192) ccw
  arc A4717 (1.0668, 2.208) -> (0.9652, 2.208) centre (1.016, 2.208) ccw
  line L2185 (1.016, 1.192) -> (-1.016, 1.192)
  arc A4718 (-1.016, 1.2428) -> (-1.016, 1.1412) centre (-1.016, 1.192) ccw
  arc A4719 (1.016, 1.1412) -> (1.016, 1.2428) centre (1.016, 1.192) ccw
  line L2186 (-1.016, 1.192) -> (-1.016, 2.208)
  arc A4720 (-0.9652, 2.208) -> (-1.0668, 2.208) centre (-1.016, 2.208) ccw
  arc A4721 (-1.0668, 1.192) -> (-0.9652, 1.192) centre (-1.016, 1.192) ccw
  line L2187 (-9.008, -1.816) -> (-9.008, 0.216)
  arc A4722 (-8.9572, 0.216) -> (-9.0588, 0.216) centre (-9.008, 0.216) ccw
  arc A4723 (-9.0588, -1.816) -> (-8.9572, -1.816) centre (-9.008, -1.816) ccw
  line L2188 (-9.008, 0.216) -> (-7.992, 0.216)
  arc A4724 (-7.992, 0.1652) -> (-7.992, 0.2668) centre (-7.992, 0.216) ccw
  arc A4725 (-9.008, 0.2668) -> (-9.008, 0.1652) centre (-9.008, 0.216) ccw
  line L2189 (-7.992, 0.216) -> (-7.992, -1.816)
  arc A4726 (-8.0428, -1.816) -> (-7.9412, -1.816) centre (-7.992, -1.816) ccw
  arc A4727 (-7.9412, 0.216) -> (-8.0428, 0.216) centre (-7.992, 0.216) ccw
  line L2190 (-7.992, -1.816) -> (-9.008, -1.816)
  arc A4728 (-9.008, -1.7652) -> (-9.008, -1.8668) centre (-9.008, -1.816) ccw
  arc A4729 (-7.992, -1.8668) -> (-7.992, -1.7652) centre (-7.992, -1.816) ccw
  line L2191 (-9.008, -3.816) -> (-9.008, -1.784)
  arc A4730 (-8.9572, -1.784) -> (-9.0588, -1.784) centre (-9.008, -1.784) ccw
  arc A4731 (-9.0588, -3.816) -> (-8.9572, -3.816) centre (-9.008, -3.816) ccw
  line L2192 (-9.008, -1.784) -> (-7.992, -1.784)
  arc A4732 (-7.992, -1.8348) -> (-7.992, -1.7332) centre (-7.992, -1.784) ccw
  arc A4733 (-9.008, -1.7332) -> (-9.008, -1.8348) centre (-9.008, -1.784) ccw
  line L2193 (-7.992, -1.784) -> (-7.992, -3.816)
  arc A4734 (-8.0428, -3.816) -> (-7.9412, -3.816) centre (-7.992, -3.816) ccw
  arc A4735 (-7.9412, -1.784) -> (-8.0428, -1.784) centre (-7.992, -1.784) ccw
  line L2194 (-7.992, -3.816) -> (-9.008, -3.816)
  arc A4736 (-9.008, -3.7652) -> (-9.008, -3.8668) centre (-9.008, -3.816) ccw
  arc A4737 (-7.992, -3.8668) -> (-7.992, -3.7652) centre (-7.992, -3.816) ccw
  line L2195 (-8.008, -1.816) -> (-8.008, 0.216)
  arc A4738 (-7.9572, 0.216) -> (-8.0588, 0.216) centre (-8.008, 0.216) ccw
  arc A4739 (-8.0588, -1.816) -> (-7.9572, -1.816) centre (-8.008, -1.816) ccw
  line L2196 (-8.008, 0.216) -> (-6.992, 0.216)
  arc A4740 (-6.992, 0.1652) -> (-6.992, 0.2668) centre (-6.992, 0.216) ccw
  arc A4741 (-8.008, 0.2668) -> (-8.008, 0.1652) centre (-8.008, 0.216) ccw
  line L2197 (-6.992, 0.216) -> (-6.992, -1.816)
  arc A4742 (-7.0428, -1.816) -> (-6.9412, -1.816) centre (-6.992, -1.816) ccw
  arc A4743 (-6.9412, 0.216) -> (-7.0428, 0.216) centre (-6.992, 0.216) ccw
  line L2198 (-6.992, -1.816) -> (-8.008, -1.816)
  arc A4744 (-8.008, -1.7652) -> (-8.008, -1.8668) centre (-8.008, -1.816) ccw
  arc A4745 (-6.992, -1.8668) -> (-6.992, -1.7652) centre (-6.992, -1.816) ccw
  line L2199 (-8.008, -3.816) -> (-8.008, -1.784)
  arc A4746 (-7.9572, -1.784) -> (-8.0588, -1.784) centre (-8.008, -1.784) ccw
  arc A4747 (-8.0588, -3.816) -> (-7.9572, -3.816) centre (-8.008, -3.816) ccw
  line L2200 (-8.008, -1.784) -> (-6.992, -1.784)
  arc A4748 (-6.992, -1.8348) -> (-6.992, -1.7332) centre (-6.992, -1.784) ccw
  arc A4749 (-8.008, -1.7332) -> (-8.008, -1.8348) centre (-8.008, -1.784) ccw
  line L2201 (-6.992, -1.784) -> (-6.992, -3.816)
  arc A4750 (-7.0428, -3.816) -> (-6.9412, -3.816) centre (-6.992, -3.816) ccw
  arc A4751 (-6.9412, -1.784) -> (-7.0428, -1.784) centre (-6.992, -1.784) ccw
  line L2202 (-6.992, -3.816) -> (-8.008, -3.816)
  arc A4752 (-8.008, -3.7652) -> (-8.008, -3.8668) centre (-8.008, -3.816) ccw
  arc A4753 (-6.992, -3.8668) -> (-6.992, -3.7652) centre (-6.992, -3.816) ccw
  line L2203 (-10.008, -0.816) -> (-10.008, 1.216)
  arc A4754 (-9.9572, 1.216) -> (-10.0588, 1.216) centre (-10.008, 1.216) ccw
  arc A4755 (-10.0588, -0.816) -> (-9.9572, -0.816) centre (-10.008, -0.816) ccw
  line L2204 (-10.008, 1.216) -> (-8.992, 1.216)
  arc A4756 (-8.992, 1.1652) -> (-8.992, 1.2668) centre (-8.992, 1.216) ccw
  arc A4757 (-10.008, 1.2668) -> (-10.008, 1.1652) centre (-10.008, 1.216) ccw
  line L2205 (-8.992, 1.216) -> (-8.992, -0.816)
  arc A4758 (-9.0428, -0.816) -> (-8.9412, -0.816) centre (-8.992, -0.816) ccw
  arc A4759 (-8.9412, 1.216) -> (-9.0428, 1.216) centre (-8.992, 1.216) ccw
  line L2206 (-8.992, -0.816) -> (-10.008, -0.816)
  arc A4760 (-10.008, -0.7652) -> (-10.008, -0.8668) centre (-10.008, -0.816) ccw
  arc A4761 (-8.992, -0.8668) -> (-8.992, -0.7652) centre (-8.992, -0.816) ccw
  line L2207 (-10.008, -2.816) -> (-10.008, -0.784)
  arc A4762 (-9.9572, -0.784) -> (-10.0588, -0.784) centre (-10.008, -0.784) ccw
  arc A4763 (-10.0588, -2.816) -> (-9.9572, -2.816) centre (-10.008, -2.816) ccw
  line L2208 (-10.008, -0.784) -> (-8.992, -0.784)
  arc A4764 (-8.992, -0.8348) -> (-8.992, -0.7332) centre (-8.992, -0.784) ccw
  arc A4765 (-10.008, -0.7332) -> (-10.008, -0.8348) centre (-10.008, -0.784) ccw
  line L2209 (-8.992, -0.784) -> (-8.992, -2.816)
  arc A4766 (-9.0428, -2.816) -> (-8.9412, -2.816) centre (-8.992, -2.816) ccw
  arc A4767 (-8.9412, -0.784) -> (-9.0428, -0.784) centre (-8.992, -0.784) ccw
  line L2210 (-8.992, -2.816) -> (-10.008, -2.816)
  arc A4768 (-10.008, -2.7652) -> (-10.008, -2.8668) centre (-10.008, -2.816) ccw
  arc A4769 (-8.992, -2.8668) -> (-8.992, -2.7652) centre (-8.992, -2.816) ccw
  line L2211 (-7.008, -3.816) -> (-7.008, -1.784)
  arc A4770 (-6.9572, -1.784) -> (-7.0588, -1.784) centre (-7.008, -1.784) ccw
  arc A4771 (-7.0588, -3.816) -> (-6.9572, -3.816) centre (-7.008, -3.816) ccw
  line L2212 (-7.008, -1.784) -> (-5.992, -1.784)
  arc A4772 (-5.992, -1.8348) -> (-5.992, -1.7332) centre (-5.992, -1.784) ccw
  arc A4773 (-7.008, -1.7332) -> (-7.008, -1.8348) centre (-7.008, -1.784) ccw
  line L2213 (-5.992, -1.784) -> (-5.992, -3.816)
  arc A4774 (-6.0428, -3.816) -> (-5.9412, -3.816) centre (-5.992, -3.816) ccw
  arc A4775 (-5.9412, -1.784) -> (-6.0428, -1.784) centre (-5.992, -1.784) ccw
  line L2214 (-5.992, -3.816) -> (-7.008, -3.816)
  arc A4776 (-7.008, -3.7652) -> (-7.008, -3.8668) centre (-7.008, -3.816) ccw
  arc A4777 (-5.992, -3.8668) -> (-5.992, -3.7652) centre (-5.992, -3.816) ccw
  line L2215 (-7.008, -5.816) -> (-7.008, -3.784)
  arc A4778 (-6.9572, -3.784) -> (-7.0588, -3.784) centre (-7.008, -3.784) ccw
  arc A4779 (-7.0588, -5.816) -> (-6.9572, -5.816) centre (-7.008, -5.816) ccw
  line L2216 (-7.008, -3.784) -> (-5.992, -3.784)
  arc A4780 (-5.992, -3.8348) -> (-5.992, -3.7332) centre (-5.992, -3.784) ccw
  arc A4781 (-7.008, -3.7332) -> (-7.008, -3.8348) centre (-7.008, -3.784) ccw
  line L2217 (-5.992, -3.784) -> (-5.992, -5.816)
  arc A4782 (-6.0428, -5.816) -> (-5.9412, -5.816) centre (-5.992, -5.816) ccw
  arc A4783 (-5.9412, -3.784) -> (-6.0428, -3.784) centre (-5.992, -3.784) ccw
  line L2218 (-5.992, -5.816) -> (-7.008, -5.816)
  arc A4784 (-7.008, -5.7652) -> (-7.008, -5.8668) centre (-7.008, -5.816) ccw
  arc A4785 (-5.992, -5.8668) -> (-5.992, -5.7652) centre (-5.992, -5.816) ccw
  line L2219 (-6.008, -0.816) -> (-6.008, 1.216)
  arc A4786 (-5.9572, 1.216) -> (-6.0588, 1.216) centre (-6.008, 1.216) ccw
  arc A4787 (-6.0588, -0.816) -> (-5.9572, -0.816) centre (-6.008, -0.816) ccw
  line L2220 (-6.008, 1.216) -> (-4.992, 1.216)
  arc A4788 (-4.992, 1.1652) -> (-4.992, 1.2668) centre (-4.992, 1.216) ccw
  arc A4789 (-6.008, 1.2668) -> (-6.008, 1.1652) centre (-6.008, 1.216) ccw
  line L2221 (-4.992, 1.216) -> (-4.992, -0.816)
  arc A4790 (-5.0428, -0.816) -> (-4.9412, -0.816) centre (-4.992, -0.816) ccw
  arc A4791 (-4.9412, 1.216) -> (-5.0428, 1.216) centre (-4.992, 1.216) ccw
  line L2222 (-4.992, -0.816) -> (-6.008, -0.816)
  arc A4792 (-6.008, -0.7652) -> (-6.008, -0.8668) centre (-6.008, -0.816) ccw
  arc A4793 (-4.992, -0.8668) -> (-4.992, -0.7652) centre (-4.992, -0.816) ccw
  line L2223 (-14.984, -0.808) -> (-17.016, -0.808)
  arc A4794 (-17.016, -0.7572) -> (-17.016, -0.8588) centre (-17.016, -0.808) ccw
  arc A4795 (-14.984, -0.8588) -> (-14.984, -0.7572) centre (-14.984, -0.808) ccw
  line L2224 (-17.016, -0.808) -> (-17.016, 0.208)
  arc A4796 (-16.9652, 0.208) -> (-17.0668, 0.208) centre (-17.016, 0.208) ccw
  arc A4797 (-17.0668, -0.808) -> (-16.9652, -0.808) centre (-17.016, -0.808) ccw
  line L2225 (-17.016, 0.208) -> (-14.984, 0.208)
  arc A4798 (-14.984, 0.1572) -> (-14.984, 0.2588) centre (-14.984, 0.208) ccw
  arc A4799 (-17.016, 0.2588) -> (-17.016, 0.1572) centre (-17.016, 0.208) ccw
  line L2226 (-14.984, 0.208) -> (-14.984, -0.808)
  arc A4800 (-15.0348, -0.808) -> (-14.9332, -0.808) centre (-14.984, -0.808) ccw
  arc A4801 (-14.9332, 0.208) -> (-15.0348, 0.208) centre (-14.984, 0.208) ccw
  line L2227 (-22.192, -20.384) -> (-22.192, -22.416)
  arc A4802 (-22.2428, -22.416) -> (-22.1412, -22.416) centre (-22.192, -22.416) ccw
  arc A4803 (-22.1412, -20.384) -> (-22.2428, -20.384) centre (-22.192, -20.384) ccw
  line L2228 (-22.192, -22.416) -> (-23.208, -22.416)
  arc A4804 (-23.208, -22.3652) -> (-23.208, -22.4668) centre (-23.208, -22.416) ccw
  arc A4805 (-22.192, -22.4668) -> (-22.192, -22.3652) centre (-22.192, -22.416) ccw
  line L2229 (-23.208, -22.416) -> (-23.208, -20.384)
  arc A4806 (-23.1572, -20.384) -> (-23.2588, -20.384) centre (-23.208, -20.384) ccw
  arc A4807 (-23.2588, -22.416) -> (-23.1572, -22.416) centre (-23.208, -22.416) ccw
  line L2230 (-23.208, -20.384) -> (-22.192, -20.384)
  arc A4808 (-22.192, -20.4348) -> (-22.192, -20.3332) centre (-22.192, -20.384) ccw
  arc A4809 (-23.208, -20.3332) -> (-23.208, -20.4348) centre (-23.208, -20.384) ccw
  line L2231 (-23.192, -20.384) -> (-23.192, -22.416)
  arc A4810 (-23.2428, -22.416) -> (-23.1412, -22.416) centre (-23.192, -22.416) ccw
  arc A4811 (-23.1412, -20.384) -> (-23.2428, -20.384) centre (-23.192, -20.384) ccw
  line L2232 (-23.192, -22.416) -> (-24.208, -22.416)
  arc A4812 (-24.208, -22.3652) -> (-24.208, -22.4668) centre (-24.208, -22.416) ccw
  arc A4813 (-23.192, -22.4668) -> (-23.192, -22.3652) centre (-23.192, -22.416) ccw
  line L2233 (-24.208, -22.416) -> (-24.208, -20.384)
  arc A4814 (-24.1572, -20.384) -> (-24.2588, -20.384) centre (-24.208, -20.384) ccw
  arc A4815 (-24.2588, -22.416) -> (-24.1572, -22.416) centre (-24.208, -22.416) ccw
  line L2234 (-24.208, -20.384) -> (-23.192, -20.384)
  arc A4816 (-23.192, -20.4348) -> (-23.192, -20.3332) centre (-23.192, -20.384) ccw
  arc A4817 (-24.208, -20.3332) -> (-24.208, -20.4348) centre (-24.208, -20.384) ccw
  line L2235 (-24.392, -24.384) -> (-24.392, -26.416)
  arc A4818 (-24.4428, -26.416) -> (-24.3412, -26.416) centre (-24.392, -26.416) ccw
  arc A4819 (-24.3412, -24.384) -> (-24.4428, -24.384) centre (-24.392, -24.384) ccw
  line L2236 (-24.392, -26.416) -> (-25.408, -26.416)
  arc A4820 (-25.408, -26.3652) -> (-25.408, -26.4668) centre (-25.408, -26.416) ccw
  arc A4821 (-24.392, -26.4668) -> (-24.392, -26.3652) centre (-24.392, -26.416) ccw
  line L2237 (-25.408, -26.416) -> (-25.408, -24.384)
  arc A4822 (-25.3572, -24.384) -> (-25.4588, -24.384) centre (-25.408, -24.384) ccw
  arc A4823 (-25.4588, -26.416) -> (-25.3572, -26.416) centre (-25.408, -26.416) ccw
  line L2238 (-25.408, -24.384) -> (-24.392, -24.384)
  arc A4824 (-24.392, -24.4348) -> (-24.392, -24.3332) centre (-24.392, -24.384) ccw
  arc A4825 (-25.408, -24.3332) -> (-25.408, -24.4348) centre (-25.408, -24.384) ccw
  line L2239 (-25.408, -24.416) -> (-25.408, -22.384)
  arc A4826 (-25.3572, -22.384) -> (-25.4588, -22.384) centre (-25.408, -22.384) ccw
  arc A4827 (-25.4588, -24.416) -> (-25.3572, -24.416) centre (-25.408, -24.416) ccw
  line L2240 (-25.408, -22.384) -> (-24.392, -22.384)
  arc A4828 (-24.392, -22.4348) -> (-24.392, -22.3332) centre (-24.392, -22.384) ccw
  arc A4829 (-25.408, -22.3332) -> (-25.408, -22.4348) centre (-25.408, -22.384) ccw
  line L2241 (-24.392, -22.384) -> (-24.392, -24.416)
  arc A4830 (-24.4428, -24.416) -> (-24.3412, -24.416) centre (-24.392, -24.416) ccw
  arc A4831 (-24.3412, -22.384) -> (-24.4428, -22.384) centre (-24.392, -22.384) ccw
  line L2242 (-24.392, -24.416) -> (-25.408, -24.416)
  arc A4832 (-25.408, -24.3652) -> (-25.408, -24.4668) centre (-25.408, -24.416) ccw
  arc A4833 (-24.392, -24.4668) -> (-24.392, -24.3652) centre (-24.392, -24.416) ccw
  line L2243 (-3.984, -1.808) -> (-6.016, -1.808)
  arc A4834 (-6.016, -1.7572) -> (-6.016, -1.8588) centre (-6.016, -1.808) ccw
  arc A4835 (-3.984, -1.8588) -> (-3.984, -1.7572) centre (-3.984, -1.808) ccw
  line L2244 (-6.016, -1.808) -> (-6.016, -0.792)
  arc A4836 (-5.9652, -0.792) -> (-6.0668, -0.792) centre (-6.016, -0.792) ccw
  arc A4837 (-6.0668, -1.808) -> (-5.9652, -1.808) centre (-6.016, -1.808) ccw
  line L2245 (-6.016, -0.792) -> (-3.984, -0.792)
  arc A4838 (-3.984, -0.8428) -> (-3.984, -0.7412) centre (-3.984, -0.792) ccw
  arc A4839 (-6.016, -0.7412) -> (-6.016, -0.8428) centre (-6.016, -0.792) ccw
  line L2246 (-3.984, -0.792) -> (-3.984, -1.808)
  arc A4840 (-4.0348, -1.808) -> (-3.9332, -1.808) centre (-3.984, -1.808) ccw
  arc A4841 (-3.9332, -0.792) -> (-4.0348, -0.792) centre (-3.984, -0.792) ccw
  line L2247 (8.992, 10.184) -> (8.992, 12.216)
  arc A4842 (9.0428, 12.216) -> (8.9412, 12.216) centre (8.992, 12.216) ccw